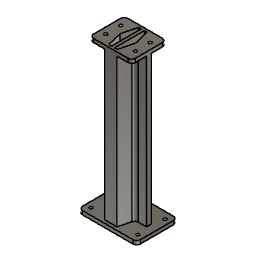
0812_arm_long v4 (Autodesk Fusion 360 design; units mm, degrees)
Autodesk Fusion 360 part; units mm, degrees
sketch "스케치1" plane through (0, 0, 0) normal (0, 0, 1) x (1, 0, 0)
  line L0 (-23.5, 16.5) -> (23.5, 16.5)
  line L1 (23.5, 16.5) -> (23.5, -16.5)
  line L2 (23.5, -16.5) -> (-23.5, -16.5)
  line L3 (-23.5, -16.5) -> (-23.5, 16.5)
  line L4 (-23.5, 0) -> (23.5, 0) construction
  line L5 (-19, 11) -> (19, 11) construction
  line L6 (19, 11) -> (19, -11) construction
  line L7 (19, -11) -> (-19, -11) construction
  line L8 (-19, -11) -> (-19, 11) construction
  line L9 (-19, 0) -> (19, 0) construction
  circle A0 centre (-19, 11) radius 1.5
  circle A1 centre (19, 11) radius 1.5
  circle A2 centre (-19, -11) radius 1.5
  circle A3 centre (19, -11) radius 1.5
  point P0 (-23.5, 0)
  point P1 (23.5, 0)
  point P2 (-19, 0)
  point P3 (19, 0)
  dimension "d1" = 47
  dimension "d2" = 33
  dimension "d3" = 38
  dimension "d4" = 22
  dimension "d5" = 3
  dimension "d6" = 3
  dimension "d7" = 3
  dimension "d8" = 3
  constraint horizontal L0
  constraint vertical L1
  constraint horizontal L2
  constraint vertical L3
  constraint midpoint L3 P0
  constraint midpoint L1 P1
  constraint coincident P0 L4.start
  constraint coincident P1 L4.end
  constraint midpoint L4 origin
  constraint horizontal L5
  constraint vertical L6
  constraint horizontal L7
  constraint vertical L8
  constraint midpoint L8 P2
  constraint midpoint L6 P3
  constraint coincident P2 L9.start
  constraint coincident P3 L9.end
  constraint midpoint L9 origin
  constraint coincident L5.start L8.end
  constraint coincident L5.end L6.start
  constraint coincident L7.end L8.start
  constraint coincident L6.end L7.start
  measures "d1" distance of L0.start L0.end
  measures "d2" distance of L0.start L2.end
  measures "d3" distance of L5.start L5.end
  measures "d4" distance of L5.start L7.end
  measures "d5" diameter of A0
  measures "d6" diameter of A1
  measures "d7" diameter of A2
  measures "d8" diameter of A3
extrude "돌출1" add sketch "스케치1" along normal blind 3 makes body 1
sketch "스케치2" plane through (0, 0, 3) normal (0, 0, 1) x (-1, 0, 0)
  circle A0 centre (19, 11) radius 1.5
  circle A1 centre (-19, 11) radius 1.5
  circle A2 centre (-19, -11) radius 1.5
  circle A3 centre (19, -11) radius 1.5
  line L0 (23.5, 16.5) -> (-23.5, 16.5)
  line L1 (-23.5, 16.5) -> (-23.5, -16.5)
  line L2 (-23.5, -16.5) -> (23.5, -16.5)
  line L3 (23.5, -16.5) -> (23.5, 16.5)
  line L4 (17, -14) -> (-17, -14)
  line L5 (-17, -14) -> (-17, 14)
  line L6 (-17, 14) -> (17, 14)
  line L7 (17, 14) -> (17, -14)
  line L8 (0, -14) -> (0, 14) construction
  line L9 (12, -6) -> (-12, -6) construction
  line L10 (-12, -6) -> (-12, 6) construction
  line L11 (-12, 6) -> (12, 6) construction
  line L12 (12, 6) -> (12, -6) construction
  line L13 (0, -6) -> (0, 6) construction
  circle A4 centre (12, -6) radius 1.5
  circle A5 centre (-12, -6) radius 1.5
  circle A6 centre (12, 6) radius 1.5
  circle A7 centre (-12, 6) radius 1.5
  line L14 (17, -2) -> (-17, -2) construction
  line L15 (-17, -2) -> (-17, 2)
  line L16 (-17, 2) -> (17, 2) construction
  line L17 (17, 2) -> (17, -2)
  line L18 (0, -2) -> (0, 2) construction
  line L19 (5, -14) -> (-5, -14)
  line L20 (-5, -14) -> (-5, 14) construction
  line L21 (-5, 14) -> (5, 14)
  line L22 (5, 14) -> (5, -14) construction
  line L23 (0, -14) -> (0, 14) construction
  line L24 (5, -14) -> (8, -2)
  line L25 (8, 2) -> (5, 14)
  line L26 (-5, 14) -> (-8, 2)
  line L27 (17, -2) -> (8, -2)
  line L28 (-8, -2) -> (-17, -2)
  line L29 (-5, -14) -> (-8, -2)
  line L30 (17, 2) -> (8, 2)
  line L31 (-8, 2) -> (-17, 2)
  line L32 (3.4384, -12) -> (-3.4384, -12)
  line L33 (-3.4384, -12) -> (-6.4384, 0)
  line L34 (-6.4384, 0) -> (-3.4384, 12)
  line L35 (-3.4384, 12) -> (3.4384, 12)
  line L36 (3.4384, 12) -> (6.4384, 0)
  line L37 (6.4384, 0) -> (3.4384, -12)
  line L38 (6.4384, 0) -> (-6.4384, 0) construction
  line L39 (0, -12) -> (0, 12) construction
  line L40 (1, -12) -> (-1, -12)
  line L41 (-1, -12) -> (-1, 12)
  line L42 (-1, 12) -> (1, 12)
  line L43 (1, 12) -> (1, -12)
  line L44 (1, 0) -> (-1, 0)
  point P0 (0, -14)
  point P1 (0, 14)
  point P2 (0, -6)
  point P3 (0, 6)
  point P4 (0, 2)
  point P5 (0, -2)
  point P6 (8, -2)
  point P7 (17, -2)
  point P8 (-8, -2)
  point P9 (-17, -2)
  point P10 (8, 2)
  point P11 (17, 2)
  point P12 (-8, 2)
  point P13 (-17, 2)
  point P14 (6.4384, 0)
  point P15 (-6.4384, 0)
  point P16 (0, -12)
  point P17 (0, 12)
  point P18 (1, 0)
  point P19 (-1, 0)
  dimension "d11" = 34
  dimension "d12" = 28
  dimension "d13" = 24
  dimension "d14" = 12
  dimension "d15" = 3
  dimension "d16" = 3
  dimension "d17" = 3
  dimension "d18" = 3
  dimension "d19" = 34
  dimension "d20" = 4
  dimension "d22" = 28
  dimension "d23" = 9
  dimension "d24" = 9
  dimension "d25" = 9
  dimension "d26" = 9
  dimension "d27" = 10
  dimension "d28" = 2
  dimension "d29" = 2
  dimension "d30" = 2
  dimension "d31" = 2
  dimension "d32" = 24
  dimension "d33" = 2
  constraint horizontal L4
  constraint vertical L5
  constraint horizontal L6
  constraint vertical L7
  constraint midpoint L4 P0
  constraint midpoint L6 P1
  constraint coincident P0 L8.start
  constraint coincident P1 L8.end
  constraint midpoint L8 origin
  constraint horizontal L9
  constraint vertical L10
  constraint horizontal L11
  constraint vertical L12
  constraint midpoint L9 P2
  constraint midpoint L11 P3
  constraint coincident P2 L13.start
  constraint coincident P3 L13.end
  constraint midpoint L13 origin
  constraint coincident L9.start L12.end
  constraint coincident L9.end L10.start
  constraint coincident L11.end L12.start
  constraint coincident L10.end L11.start
  constraint horizontal L14
  constraint vertical L15
  constraint horizontal L16
  constraint vertical L17
  constraint midpoint L16 P4
  constraint midpoint L14 P5
  constraint coincident P5 L18.start
  constraint coincident P4 L18.end
  constraint midpoint L18 origin
  constraint horizontal L19
  constraint vertical L20
  constraint horizontal L21
  constraint vertical L22
  constraint midpoint L19 P0
  constraint midpoint L21 P1
  constraint midpoint L23 origin
  constraint coincident L14 P6
  constraint coincident P7 L14.start
  constraint coincident L14 P8
  constraint coincident P9 L14.end
  constraint coincident L16 P10
  constraint coincident P11 L16.end
  constraint coincident L16 P12
  constraint coincident P13 L15.end
  constraint coincident P6 L24.end
  constraint coincident P10 L25.start
  constraint coincident P12 L26.end
  constraint coincident P8 L28.start
  constraint horizontal L32
  constraint parallel L32 L35
  constraint coincident P14 L36.end
  constraint coincident P15 L33.end
  constraint horizontal L38
  constraint midpoint L38 origin
  constraint midpoint L32 P16
  constraint midpoint L35 P17
  constraint coincident P16 L39.start
  constraint coincident P17 L39.end
  constraint parallel L29 L33
  constraint collinear L23 L39
  constraint parallel L26 L34
  constraint horizontal L40
  constraint vertical L41
  constraint horizontal L42
  constraint vertical L43
  constraint midpoint L43 P18
  constraint midpoint L41 P19
  constraint coincident P18 L44.start
  constraint coincident P19 L44.end
  constraint midpoint L44 origin
  measures "d11" distance of L4.start L4.end
  measures "d12" distance of L4.start L6.end
  measures "d13" distance of L9.start L9.end
  measures "d14" distance of L9.start L11.end
  measures "d15" diameter of A4
  measures "d16" diameter of A5
  measures "d17" diameter of A6
  measures "d18" diameter of A7
  measures "d19" distance of P7 P9
  measures "d20" distance of P7 P11
  measures "d22" distance of L19.start L21.end
  measures "d23" distance of P6 P7
  measures "d24" distance of P8 P9
  measures "d25" distance of P10 P11
  measures "d26" distance of P12 P13
  measures "d27" distance of L19.start L19.end
  measures "d28" distance of L19 L32
  measures "d29" distance of L29 L33
  measures "d30" distance of L21 L35
  measures "d31" distance of L24 L37
  measures "d32" distance of L40.end L41.end
  measures "d33" distance of L40.start L40.end
extrude "돌출2" add sketch "스케치2" along normal blind 123 separate body contours L4 L5 L6 L7 L15 L17 L19 L21 L24 L25 L26 L27 L28 L29 L30 L31 | L32 L40 L41 L43 L44 | L35 L41 L42 L43 L44 makes body 2
sketch "스케치3" plane through (0, 0, 3) normal (0, 0, 1) x (-1, 0, 0)
  line L0 (17, -14) -> (-17, -14)
  line L1 (-17, -14) -> (-17, 14)
  line L2 (-17, 14) -> (17, 14)
  line L3 (17, 14) -> (17, -14)
  circle A0 centre (12, -6) radius 1.5
  circle A1 centre (-12, -6) radius 1.5
  circle A2 centre (12, 6) radius 1.5
  circle A3 centre (-12, 6) radius 1.5
  circle A4 centre (12, -6) radius 1.5
  circle A5 centre (-12, -6) radius 1.5
  circle A6 centre (-12, 6) radius 1.5
  circle A7 centre (12, 6) radius 1.5
  point P0 (17, -14)
  point P1 (-17, -14)
  point P2 (17, 14)
  point P3 (-17, 14)
  point P4 (17, -14)
  point P5 (-17, -14)
  point P6 (17, 14)
  point P7 (-17, 14)
  point P8 (12, -6)
  point P9 (-12, -6)
  point P10 (-12, 6)
  point P11 (12, 6)
  point P12 (5, -14)
  point P13 (8, -2)
  point P14 (17, -2)
  point P15 (17, 2)
  point P16 (5, -14)
  point P17 (8, -2)
  point P18 (17, -2)
  point P19 (17, 2)
  point P20 (5, 14)
  point P21 (8, 2)
  point P22 (-5, 14)
  point P23 (-8, 2)
  point P24 (8, 2)
  point P25 (5, 14)
  point P26 (-5, 14)
  point P27 (-8, 2)
  point P28 (-5, -14)
  point P29 (-8, -2)
  point P30 (-17, -2)
  point P31 (-17, 2)
  point P32 (-8, -2)
  point P33 (-5, -14)
  point P34 (-17, -2)
  point P35 (-17, 2)
  constraint coincident P4 P0
  constraint coincident P5 P1
  constraint coincident P6 P2
  constraint coincident P7 P3
  constraint horizontal L0
  constraint vertical L1
  constraint horizontal L2
  constraint vertical L3
  constraint equal A0 A4
  constraint coincident P8 A0.centre
  constraint equal A1 A5
  constraint coincident P9 A1.centre
  constraint equal A3 A6
  constraint coincident P10 A3.centre
  constraint equal A2 A7
  constraint coincident P11 A2.centre
  constraint coincident P16 P12
  constraint coincident P17 P13
  constraint coincident P18 P14
  constraint coincident P19 P15
  constraint coincident P24 P21
  constraint coincident P25 P20
  constraint coincident P26 P22
  constraint coincident P27 P23
  constraint coincident P32 P29
  constraint coincident P33 P28
  constraint coincident P34 P30
  constraint coincident P35 P31
extrude "돌출4" add sketch "스케치2" along normal blind 3 from surface at 120 contours L4 L7 L24 L27 | L4 L5 L28 L29 | L6 L7 L25 L30 | L5 L6 L26 L31 bodies 2
combine "결합1" operation add target body 1 tool bodies 2
fillet "모깎기1" radius 3 4 edges at (-17, 14, 124.5) (-17, -14, 124.5) (17, -14, 124.5) (17, 14, 124.5) on bodies 1
fillet "모깎기2" radius 3 4 edges at (23.5, 16.5, 1.5) (-23.5, 16.5, 1.5) (-23.5, -16.5, 1.5) (23.5, -16.5, 1.5) on bodies 1
fillet "모깎기3" radius 3 4 edges at (-8, 2, 63) (-8, -2, 63) (8, -2, 63) (8, 2, 63) on bodies 1
thread "스레드1" "ISO Metric profile 3.0 M3x0.5 6H" major diameter 3.086 minor diameter 2.529 pitch 0.5 angle 60 resizes the face on face at (10.5019, 6.0748, 125) on bodies 1
thread "스레드2" "ISO Metric profile 3.0 M3x0.5 6H" major diameter 3.086 minor diameter 2.529 pitch 0.5 angle 60 resizes the face on face at (10.5019, -6.0748, 124) on bodies 1
thread "스레드3" "ISO Metric profile 3.0 M3x0.5 6H" major diameter 3.086 minor diameter 2.529 pitch 0.5 angle 60 resizes the face on face at (-13.4981, 5.9252, 124) on bodies 1
thread "스레드4" "ISO Metric profile 3.0 M3x0.5 6H" major diameter 3.086 minor diameter 2.529 pitch 0.5 angle 60 resizes the face on face at (-13.4981, -6.0748, 124) on bodies 1
thread "스레드5" "ISO Metric profile 3.0 M3x0.5 6H" major diameter 3.086 minor diameter 2.529 pitch 0.5 angle 60 resizes the face on face at (-17.5019, 11.0748, 1) on bodies 1
thread "스레드6" "ISO Metric profile 3.0 M3x0.5 6H" major diameter 3.086 minor diameter 2.529 pitch 0.5 angle 60 resizes the face on face at (-17.5019, -10.9252, 1) on bodies 1
thread "스레드7" "ISO Metric profile 3.0 M3x0.5 6H" major diameter 3.086 minor diameter 2.529 pitch 0.5 angle 60 resizes the face on face at (20.4981, 11.0748, 1) on bodies 1
thread "스레드8" "ISO Metric profile 3.0 M3x0.5 6H" major diameter 3.086 minor diameter 2.529 pitch 0.5 angle 60 resizes the face on face at (20.4981, -10.9252, 1) on bodies 1
sketch "스케치4" plane through (0, 0, 0) normal (0, 0, 1) x (1, 0, 0)
  line L0 (-1.25, 14) -> (1.25, 14)
  line L1 (1.25, 14) -> (1.25, -14)
  line L2 (1.25, -14) -> (-1.25, -14)
  line L3 (-1.25, -14) -> (-1.25, 14)
  line L4 (-1.25, 0) -> (1.25, 0) construction
  point P0 (1.25, 0)
  point P1 (-1.25, 0)
  dimension "d48" = 2.5
  dimension "d49" = 28
  constraint horizontal L0
  constraint vertical L1
  constraint horizontal L2
  constraint vertical L3
  constraint midpoint L1 P0
  constraint midpoint L3 P1
  constraint coincident P1 L4.start
  constraint coincident P0 L4.end
  constraint midpoint L4 origin
  measures "d48" distance of L0.start L0.end
  measures "d49" distance of L0.end L1.end
extrude "돌출5" add sketch "스케치4" along normal blind 126 separate body makes body 3
combine "결합2" operation add target body 1 tool bodies 3
extrude "돌출3" [rolled back] profile offset 120 along distance 3 taper angle 0
